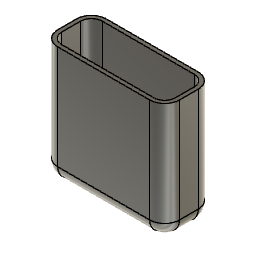
mucon_v2.6 (Autodesk Fusion 360 design; units mm, degrees)
Autodesk Fusion 360 part; units mm, degrees
sketch "スケッチ1" plane through (0, 0, 0) normal (0, 0, 1) x (1, 0, 0)
  line L0 (12.3, -4.9) -> (-12.3, -4.9)
  line L1 (-12.3, -4.9) -> (-12.3, 4.9)
  line L2 (-12.3, 4.9) -> (12.3, 4.9)
  line L3 (12.3, 4.9) -> (12.3, -4.9)
  line L4 (12.3, -4.9) -> (-12.3, 4.9) construction
  line L5 (-12.3, -4.9) -> (12.3, 4.9) construction
  dimension "d1" = 24.6
  dimension "d2" = 9.8
  constraint horizontal L0
  constraint perpendicular L0 L1
  constraint parallel L0 L2
  constraint parallel L1 L3
  constraint coincident L4 origin
  constraint coincident L5 origin
  measures "d1" distance of L1.end L2.end
  measures "d2" distance of L0.end L1.end
extrude "押し出し1" add sketch "スケッチ1" along normal blind 24
fillet "フィレット2" radius 3 8 edges at (0, -4.9, 0) (12.3, 0, 0) (0, 4.9, 0) (-12.3, 0, 0) (12.3, -4.9, 12) (-12.3, -4.9, 12) (-12.3, 4.9, 12) (12.3, 4.9, 12)
shell "シェル2" thickness 0.8 removed faces 1 at (3.1, -1.6333, 24)
